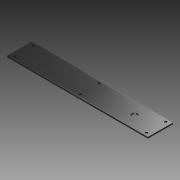
# Autodesk Inventor part: EnclosurePanelBottomFront
Saved by Autodesk Inventor 2016 (Build 200138000, 138)
## iProperties
Category: Panel
Created: 2015-01-12
Part Number: EnclosurePanelBottomFront
Material: ABS Plastic
Document SubType Name: Modeling
Designer: Jack
Density: 1.06 g/cm^3
Appearance: Smooth - Dark Gray
Mass: 203.72 g
Surface Area: 867.916 cm^2
Volume: 192.189 cm^3
Author: Jack
Title: Enclosure Bottom Panel
Autodesk Inventor part; units mm, degrees
ref_plane "YZ Plane" through (0, 0, 0) normal (1, 0, 0) x (0, 1, 0)
ref_plane "XZ Plane" through (0, 0, 0) normal (0, 1, 0) x (-1, 0, 0)
ref_plane "XY Plane" through (0, 0, 0) normal (0, 0, 1) x (1, 0, 0)
sketch "Sketch1" plane through (0, 0, 0) normal (0, 0, 1) x (1, 0, 0)
  line L0 (0, 0) -> (479.525, 0)
  line L1 (479.525, 0) -> (479.525, 85)
  line L2 (479.525, 85) -> (0, 85)
  line L3 (0, 85) -> (0, 0)
  dimension "d0" = 479.525
  dimension "d1" = 85
  constraints: 8 end point, 2 parallel, 1 horizontal, 1 perpendicular
  measures "d0" distance of L2.end L1.end
  measures "d1" distance of L2.end L0.start
extrude "Extrusion1" add sketch "Sketch1" along normal blind 4.7625
sketch "Sketch2" plane through (0, 0, 4.7625) normal (0, 0, 1) x (1, 0, 0)
  line L0 (0, 0) -> (479.525, 0) projected
  line L1 (382.925, 46.859) -> (382.925, 38.141)
  line L2 (399.525, 38.141) -> (399.525, 46.859)
  arc A0 (382.925, 38.141) -> (399.525, 38.141) centre (391.225, 42.5) ccw
  arc A1 (399.525, 46.859) -> (382.925, 46.859) centre (391.225, 42.5) ccw
  line L3 (479.525, 0) -> (479.525, 85) projected
  dimension "d5" = 16.6
  dimension "d6" = 9.375
  dimension "d7" = 9.375
  dimension "d8" = 42.5
  dimension "d23" = 80
  constraints: 4 end point, 4 point on circle, 2 centre point, 2 parallel, 1 vertical
  measures "d5" distance between parallel lines of L1 L2
  measures "d6" radius of A1
  measures "d7" radius of A0
  measures "d8" distance from line of L0 A0.centre
  measures "d23" distance between parallel lines of L3 L2
extrude "Extrusion2" cut sketch "Sketch2" against normal up to next
sketch "Sketch3" plane through (0, 0, 4.7625) normal (0, 0, 1) x (1, 0, 0)
  line L0 (0, 0) -> (479.525, 0) projected
  line L1 (479.525, 0) -> (479.525, 85) projected
  line L2 (479.525, 85) -> (0, 85) projected
  line L3 (0, 85) -> (0, 0) projected
  circle A0 centre (14.7625, 75) radius 2.25
  circle A1 centre (14.7625, 10) radius 2.25
  circle A2 centre (464.7625, 75) radius 2.25
  circle A3 centre (464.7625, 10) radius 2.25
  circle A4 centre (238.2625, 10) radius 2.25
  circle A5 centre (238.2625, 75) radius 2.25
  dimension "d12" = 4.5
  dimension "d13" = 14.7625
  dimension "d14" = 14.7625
  dimension "d15" = 10
  dimension "d16" = 10
  dimension "d17" = 241.2625
  constraints: 6 centre point, 5 equal radius, 4 horizontal alignment, 3 vertical alignment
  measures "d12" diameter of A0
  measures "d13" distance from line of L3 A0.centre
  measures "d14" distance from line of L1 A2.centre
  measures "d15" distance from line of L0 A1.centre
  measures "d16" distance from line of L2 A0.centre
  measures "d17" distance from line of L1 A4.centre
extrude "Extrusion3" cut sketch "Sketch3" against normal up to next contours A0 | A1 | A2 | A3 | A4 | A5
chamfer "Chamfer1" distance 2 angle 45 6 edges at (236.0125, 75, 4.7625) (236.0125, 10, 4.7625) (462.5125, 10, 4.7625) (462.5125, 75, 4.7625) (12.5125, 75, 4.7625) (12.5125, 10, 4.7625)
body "Solid1"
